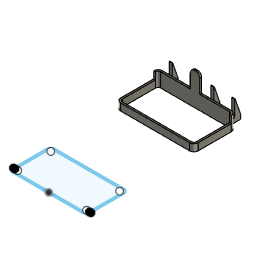
BirdBoxHolder Attempt 0 v1 (Autodesk Fusion 360 design; units mm, degrees)
Autodesk Fusion 360 part; units mm, degrees
sketch "SizeOfTheBoxToHold" plane through (0, 0, 0) normal (0, 0, 1) x (1, 0, 0)
  line L0 (2.5, 0) -> (70.8, 0)
  line L1 (73.3, 2.5) -> (73.3, 35.3)
  line L2 (70.8, 37.8) -> (2.5, 37.8)
  line L3 (0, 35.3) -> (0, 2.5)
  arc A0 (2.5, 37.8) -> (0, 35.3) centre (2.5, 35.3) ccw
  arc A1 (73.3, 35.3) -> (70.8, 37.8) centre (70.8, 35.3) ccw
  arc A2 (70.8, 0) -> (73.3, 2.5) centre (70.8, 2.5) ccw
  arc A3 (0, 2.5) -> (2.5, 0) centre (2.5, 2.5) ccw
  point P0 (73.3, 0)
  point P1 (0, 37.8)
  dimension "d1" = 73.3
  dimension "d2" = 37.8
  dimension "d3" = 2.5
  dimension "d4" = 2.5
  constraint horizontal L0
  constraint vertical L1
  constraint horizontal L2
  constraint vertical L3
  constraint coincident P1 L3
  constraint coincident P1 L2
  constraint tangent L3 A0
  constraint tangent L2 A0
  constraint tangent L2 A1
  constraint tangent L1 A1
  constraint coincident P0 L1
  constraint coincident P0 L0
  constraint tangent L1 A2
  constraint tangent L0 A2
  constraint equal A1 A2
  constraint coincident origin L0
  constraint coincident origin L3
  constraint tangent L0 A3
  constraint tangent L3 A3
  constraint equal A1 A3
  measures "d1" distance of origin P0
  measures "d2" distance of origin P1
  measures "d3" radius of A0
  measures "d4" radius of A1
sketch "Border of Box" plane through (0, 0, 0) normal (0, 0, 1) x (1, 0, 0)
  line L0 (0, 35.3) -> (0, 2.5)
  arc A0 (0, 2.5) -> (2.5, 0) centre (2.5, 2.5) ccw
  line L1 (2.5, 0) -> (70.8, 0)
  arc A1 (70.8, 0) -> (73.3, 2.5) centre (70.8, 2.5) ccw
  line L2 (73.3, 2.5) -> (73.3, 35.3)
  arc A2 (73.3, 35.3) -> (70.8, 37.8) centre (70.8, 35.3) ccw
  line L3 (70.8, 37.8) -> (2.5, 37.8)
  arc A3 (2.5, 37.8) -> (0, 35.3) centre (2.5, 35.3) ccw
  line L4 (70.8, 39.6) -> (2.5, 39.6)
  arc A4 (2.5, 39.6) -> (-1.8, 35.3) centre (2.5, 35.3) ccw
  line L5 (-1.8, 35.3) -> (-1.8, 2.5)
  arc A5 (-1.8, 2.5) -> (2.5, -1.8) centre (2.5, 2.5) ccw
  line L6 (2.5, -1.8) -> (70.8, -1.8)
  arc A6 (70.8, -1.8) -> (75.1, 2.5) centre (70.8, 2.5) ccw
  line L7 (75.1, 2.5) -> (75.1, 35.3)
  arc A7 (75.1, 35.3) -> (70.8, 39.6) centre (70.8, 35.3) ccw
  dimension "d5" = 2.5
  dimension "d6" = 2.5
  dimension "d7" = 1.8
  constraint horizontal L1
  constraint vertical L2
  constraint horizontal L3
  constraint vertical L0
  constraint tangent L0 A3
  constraint tangent L3 A3
  constraint tangent A2 L3
  constraint tangent L2 A2
  constraint tangent A1 L2
  constraint tangent L1 A1
  constraint equal A1 A2
  constraint tangent A0 L1
  constraint tangent L0 A0
  constraint equal A0 A2
  measures "d5" radius of A3
  measures "d6" radius of A2
extrude "Extrude1" add sketch "Border of Box" against normal blind 7 makes body 1
sketch "Hook On side" plane through (0, 0, 0) normal (1, 0, 0) x (0, 1, 0)
  line L0 (0, 0) -> (-12.8, 0)
  line L1 (-13, -0.2) -> (-13, -3.9528)
  line L2 (-5.0424, -4) -> (0, -4)
  line L3 (0, -4) -> (0, 0)
  line L4 (-12.9892, -4.0176) -> (-7.4316, -20.2395)
  line L5 (-7.0424, -20.1747) -> (-7.0424, -6)
  arc A0 (-6.8424, -4) -> (-7.0424, -4.2) centre (-6.8424, -4.2) ccw
  arc A1 (-12.8, 0) -> (-13, -0.2) centre (-12.8, -0.2) ccw
  arc A2 (-13, -3.9528) -> (-12.9892, -4.0176) centre (-12.8, -3.9528) ccw
  arc A3 (-7.4316, -20.2395) -> (-7.0424, -20.1747) centre (-7.2424, -20.1747) ccw
  arc A4 (-5.0424, -4) -> (-7.0424, -6) centre (-5.0424, -6) ccw
  dimension "d10" = 0.2
  dimension "d11" = 2
  constraint horizontal L0
  constraint vertical L1
  constraint horizontal L2
  constraint vertical L3
  constraint coincident L0.start L3.end
  constraint perpendicular L2 L5
  constraint tangent L2 A0
  constraint tangent L5 A0
  constraint tangent L0 A1
  constraint tangent L1 A1
  constraint equal A0 A1
  constraint tangent L1 A2
  constraint tangent L4 A2
  constraint equal A0 A2
  constraint tangent L4 A3
  constraint tangent L5 A3
  constraint equal A0 A3
  constraint coincident L5 A0.end
  constraint coincident L2 A0.start
  constraint tangent L5 A4
  constraint tangent L2 A4
  measures "d10" radius of A0
  measures "d11" radius of A4
sketch "Sketch4" plane through (0, 0, 0) normal (0, 0, 1) x (1, 0, 0)
  line L0 (73.3, 2.5) -> (75.1, 2.5)
  line L1 (-1.8, 2.5) -> (0, 2.5)
  arc A0 (70.8, 0) -> (73.3, 2.5) centre (70.8, 2.5) ccw
  line L2 (73.3, 2.5) -> (73.3, 35.3)
  arc A1 (73.3, 35.3) -> (70.8, 37.8) centre (70.8, 35.3) ccw
  line L3 (70.8, 37.8) -> (2.5, 37.8)
  arc A2 (2.5, 37.8) -> (0, 35.3) centre (2.5, 35.3) ccw
  line L4 (0, 35.3) -> (0, 2.5)
  arc A3 (0, 2.5) -> (2.5, 0) centre (2.5, 2.5) ccw
  line L5 (2.5, 0) -> (70.8, 0)
  arc A4 (70.8, -1.8) -> (75.1, 2.5) centre (70.8, 2.5) ccw
  line L6 (75.1, 2.5) -> (75.1, 35.3)
  arc A5 (75.1, 35.3) -> (70.8, 39.6) centre (70.8, 35.3) ccw
  line L7 (70.8, 39.6) -> (2.5, 39.6)
  arc A6 (2.5, 39.6) -> (-1.8, 35.3) centre (2.5, 35.3) ccw
  line L8 (-1.8, 35.3) -> (-1.8, 2.5)
  arc A7 (-1.8, 2.5) -> (2.5, -1.8) centre (2.5, 2.5) ccw
  line L9 (2.5, -1.8) -> (70.8, -1.8)
  line L10 (36.65, -1.8) -> (36.65, 0)
  line L11 (32, 0) -> (41.3, 0)
  line L12 (41.3, 0) -> (41.3, -1.8)
  line L13 (41.3, -1.8) -> (32, -1.8)
  line L14 (32, -1.8) -> (32, 0)
  line L15 (32, 0) -> (41.3, -1.8) construction
  line L16 (41.3, 0) -> (32, -1.8) construction
  point P0 (73.3, 2.5)
  point P1 (75.1, 2.5)
  point P2 (-1.8, 2.5)
  point P3 (0, 2.5)
  point P4 (36.65, -0.9)
  dimension "d12" = 2.5
  dimension "d13" = 2.5
  constraint coincident P0 L0.start
  constraint coincident P1 L0.end
  constraint coincident P2 L1.start
  constraint coincident P3 L1.end
  constraint horizontal L5
  constraint vertical L2
  constraint horizontal L3
  constraint vertical L4
  constraint tangent A2 L4
  constraint tangent L3 A2
  constraint tangent A1 L3
  constraint tangent L2 A1
  constraint tangent A0 L2
  constraint tangent A0 L5
  constraint equal A0 A1
  constraint tangent A3 L5
  constraint tangent L4 A3
  constraint equal A1 A3
  constraint midpoint L9 L10.start
  constraint midpoint L5 L10.end
  constraint horizontal L11
  constraint perpendicular L11 L12
  constraint parallel L11 L13
  constraint parallel L12 L14
  constraint coincident L15 P4
  constraint coincident L16 P4
  constraint coincident L5 L11.start
  constraint midpoint L10 P4
  measures "d12" radius of A2
  measures "d13" radius of A1
extrude "Extrude2" add sketch "Sketch4" against normal blind 14 contours L0 A0 L5 A4 L9 L12 | L5 L9 L10 L11 L12 L13 | L5 L9 L10 L11 L13 L14 | L1 A3 L5 A7 L9 L14 bodies 1
extrude "Extrude3" add sketch "Hook On side" along normal blind 3 separate body makes body 2
move_body "Move1" bodies 2 to x (1, 0, 0) y (0, 1, 0) z (0, 0, 1) at (4, 0, 0)
pattern_linear "R-Pattern1" count 4 spacing 20.6667 along (1, 0, 0) of bodies 2 makes body 3 at (24.6667, -9.1544, -10.0857) makes body 4 at (45.3333, -9.1544, -10.0857) makes body 5 at (66, -9.1544, -10.0857)
extrude "Extrude4" add sketch "Sketch4" against normal blind 32 contours L5 L9 L10 L11 L12 L13 | L5 L9 L10 L11 L13 L14 bodies 1
fillet "Fillet1" radius 4 2 edges at (32, -0.9, -32) (41.3, -0.9, -32) on bodies 1
combine "Combine1" operation add target body 1 tool bodies 2 5 3 4
copy_body "CopyPasteBodies1" bodies 1 makes body 6
move_body "Move2" bodies 6 to x (1, 0, 0) y (0, -1, 0) z (0, 0, -1) at (0, 144.2, 0)
hidden bodies 1
named bodies: "Bird FoodBox Holder", "Bird FoodBox Holder Print Direction"
